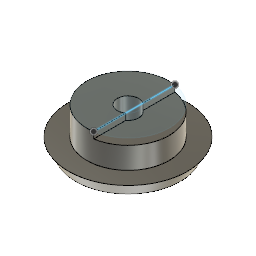
bar end spacer v4 (Autodesk Fusion 360 design; units mm, degrees)
Autodesk Fusion 360 part; units mm, degrees
sketch "Sketch1" plane through (0, 0, 0) normal (0, 0, 1) x (1, 0, 0)
  circle A0 centre (0, 0) radius 11
  circle A1 centre (0, 0) radius 2.85
  dimension "d1" = 22
  dimension "d2" = 5.7
  constraint coincident A0.centre A1.centre
  constraint concentric A0 A1
  measures "d1" diameter of A0
  measures "d2" diameter of A1
extrude "Extrude1" add sketch "Sketch1" along normal blind 7.5
sketch "Sketch2" plane through (0, 0, 7.5) normal (0, 0, 1) x (-1, 0, 0)
  circle A0 centre (0, 0) radius 2.85
  circle A1 centre (0, 0) radius 11
  line L0 (-1.6821, -10.8706) -> (-1.6821, 10.8706)
  constraint coincident A1 L0.start
  constraint coincident A1 L0.end
  constraint vertical L0
extrude "Extrude2" cut sketch "Sketch2" against normal blind 1.7 contours A0 A1 L0 picked at (-5.1344, 6.4731)
sketch "Sketch3" plane through (0, 0, 0) normal (0, 0, -1) x (1, 0, 0)
  circle A0 centre (0, 0) radius 2.85
  circle A1 centre (0, 0) radius 11
  circle A2 centre (0, 0) radius 14
  dimension "d7" = 28
  constraint coincident A0.centre A1.centre
  measures "d7" diameter of A2
extrude "Extrude3" add sketch "Sketch3" against normal blind 3.4 draft 30 from surface at 3.4 contours A1 | A2
extrude "Extrude4" cut sketch "Sketch2" against normal up to surface (10.9 mm away) contours A0 L0 | A0 L0
named bodies: "bar end spacer"
